Autodesk Fusion 360 part; units mm, degrees
(part 2 of 2)
sketch "Sketch4" plane through (0, 66.2073, 0) normal (0, 1, 0) x (-1, 0, 0)
  line L0 (-39.5671, 5.0322) -> (-39.5671, 0)
  line L1 (-39.5671, 0) -> (-35, 0)
  line L2 (-35, 0) -> (-35, 30)
  line L3 (-35, 30) -> (-45.5671, 30)
  line L4 (-45.5671, 30) -> (-45.5671, 5.0322)
  line L5 (-45.5671, 5.0322) -> (-39.5671, 5.0322)
  line L6 (-39.5671, 5.0322) -> (-19, 5.0322)
  line L7 (-19, 5.0322) -> (-19, 0)
  line L8 (-19, 0) -> (-39.5671, 0)
  line L9 (-39.5671, 0) -> (-39.5671, 5.0322)
  line L10 (-45.5671, 29) -> (-45.5671, 19)
  line L11 (-45.5671, 18.6501) -> (-45.5671, 13.7057)
  line L12 (-45.5671, 13.3545) -> (-45.5671, 9.6128)
  line L13 (-45, 29) -> (-44, 29)
  line L14 (-44, 29) -> (-44, 19)
  line L15 (-44, 19) -> (-45, 19)
  line L16 (-45, 19) -> (-45, 29)
  line L17 (-43.5, 29) -> (-43, 29)
  line L18 (-43, 29) -> (-43, 19)
  line L19 (-43, 19) -> (-43.5, 19)
  line L20 (-43.5, 19) -> (-43.5, 29)
  line L21 (-42.625, 19) -> (-42.625, 29)
  line L22 (-42.125, 29) -> (-42.125, 19)
  line L23 (-42.625, 29) -> (-42.125, 29)
  line L24 (-42.125, 19) -> (-42.625, 19)
  line L25 (-41.75, 19) -> (-41.75, 29)
  line L26 (-41.25, 29) -> (-41.25, 19)
  line L27 (-41.75, 29) -> (-41.25, 29)
  line L28 (-41.25, 19) -> (-41.75, 19)
  line L29 (-40.875, 19) -> (-40.875, 29)
  line L30 (-40.375, 29) -> (-40.375, 19)
  line L31 (-40.875, 29) -> (-40.375, 29)
  line L32 (-40.375, 19) -> (-40.875, 19)
  line L33 (-40, 19) -> (-40, 29)
  line L34 (-39.5, 29) -> (-39.5, 19)
  line L35 (-40, 29) -> (-39.5, 29)
  line L36 (-39.5, 19) -> (-40, 19)
  line L37 (-39.125, 19) -> (-39.125, 29)
  line L38 (-38.625, 29) -> (-38.625, 19)
  line L39 (-39.125, 29) -> (-38.625, 29)
  line L40 (-38.625, 19) -> (-39.125, 19)
  line L41 (-38.25, 19) -> (-38.25, 29)
  line L42 (-37.75, 29) -> (-37.75, 19)
  line L43 (-38.25, 29) -> (-37.75, 29)
  line L44 (-37.75, 19) -> (-38.25, 19)
  line L45 (-37.375, 19) -> (-37.375, 29)
  line L46 (-36.875, 29) -> (-36.875, 19)
  line L47 (-37.375, 29) -> (-36.875, 29)
  line L48 (-36.875, 19) -> (-37.375, 19)
  line L49 (-36.5, 19) -> (-36.5, 29)
  line L50 (-36, 29) -> (-36, 19)
  line L51 (-36.5, 29) -> (-36, 29)
  line L52 (-36, 19) -> (-36.5, 19)
  line L53 (-40.8767, 18.5179) -> (-40.3767, 18.5179)
  line L54 (-40.3767, 18.5179) -> (-40.3767, 10.3968)
  line L55 (-40.3767, 10.3968) -> (-40.8767, 10.3968)
  line L56 (-40.8767, 10.3968) -> (-40.8767, 18.5179)
  line L57 (-39.4967, 18.5179) -> (-39.4967, 10.3968)
  line L58 (-39.9967, 10.3968) -> (-39.9967, 18.5179)
  line L59 (-39.9967, 18.5179) -> (-39.4967, 18.5179)
  line L60 (-39.4967, 10.3968) -> (-39.9967, 10.3968)
  line L61 (-38.6167, 18.5179) -> (-38.6167, 10.3968)
  line L62 (-39.1167, 10.3968) -> (-39.1167, 18.5179)
  line L63 (-39.1167, 18.5179) -> (-38.6167, 18.5179)
  line L64 (-38.6167, 10.3968) -> (-39.1167, 10.3968)
  line L65 (-37.7367, 18.5179) -> (-37.7367, 10.3968)
  line L66 (-38.2367, 10.3968) -> (-38.2367, 18.5179)
  line L67 (-38.2367, 18.5179) -> (-37.7367, 18.5179)
  line L68 (-37.7367, 10.3968) -> (-38.2367, 10.3968)
  line L69 (-36.8567, 18.5179) -> (-36.8567, 10.3968)
  line L70 (-37.3567, 10.3968) -> (-37.3567, 18.5179)
  line L71 (-37.3567, 18.5179) -> (-36.8567, 18.5179)
  line L72 (-36.8567, 10.3968) -> (-37.3567, 10.3968)
  line L73 (-35.9767, 18.5179) -> (-35.9767, 10.3968)
  line L74 (-36.4767, 10.3968) -> (-36.4767, 18.5179)
  line L75 (-36.4767, 18.5179) -> (-35.9767, 18.5179)
  line L76 (-35.9767, 10.3968) -> (-36.4767, 10.3968)
  line L77 (-35.0392, 18.5179) -> (-35.0392, 10.3968)
  line L78 (-35.5392, 10.3968) -> (-35.5392, 18.5179)
  line L79 (-35.5392, 18.5179) -> (-35.0392, 18.5179)
  line L80 (-35.0392, 10.3968) -> (-35.5392, 10.3968)
  line L81 (-34.1017, 18.5179) -> (-34.1017, 10.3968)
  line L82 (-34.6017, 10.3968) -> (-34.6017, 18.5179)
  line L83 (-34.6017, 18.5179) -> (-34.1017, 18.5179)
  line L84 (-34.1017, 10.3968) -> (-34.6017, 10.3968)
  line L85 (-33.1642, 18.5179) -> (-33.1642, 10.3968)
  line L86 (-33.6642, 10.3968) -> (-33.6642, 18.5179)
  line L87 (-33.6642, 18.5179) -> (-33.1642, 18.5179)
  line L88 (-33.1642, 10.3968) -> (-33.6642, 10.3968)
  line L89 (-32.2267, 18.5179) -> (-32.2267, 10.3968)
  line L90 (-32.7267, 10.3968) -> (-32.7267, 18.5179)
  line L91 (-32.7267, 18.5179) -> (-32.2267, 18.5179)
  line L92 (-32.2267, 10.3968) -> (-32.7267, 10.3968)
  line L93 (-31.2892, 18.5179) -> (-31.2892, 10.3968)
  line L94 (-31.7892, 10.3968) -> (-31.7892, 18.5179)
  line L95 (-31.7892, 18.5179) -> (-31.2892, 18.5179)
  line L96 (-31.2892, 10.3968) -> (-31.7892, 10.3968)
  line L97 (-30.3517, 18.5179) -> (-30.3517, 10.3968)
  line L98 (-30.8517, 10.3968) -> (-30.8517, 18.5179)
  line L99 (-30.8517, 18.5179) -> (-30.3517, 18.5179)
  line L100 (-30.3517, 10.3968) -> (-30.8517, 10.3968)
  line L101 (-29.4142, 18.5179) -> (-29.4142, 10.3968)
  line L102 (-29.9142, 10.3968) -> (-29.9142, 18.5179)
  line L103 (-29.9142, 18.5179) -> (-29.4142, 18.5179)
  line L104 (-29.4142, 10.3968) -> (-29.9142, 10.3968)
  line L105 (-28.4767, 18.5179) -> (-28.4767, 10.3968)
  line L106 (-28.9767, 10.3968) -> (-28.9767, 18.5179)
  line L107 (-28.9767, 18.5179) -> (-28.4767, 18.5179)
  line L108 (-28.4767, 10.3968) -> (-28.9767, 10.3968)
  line L109 (-27.5392, 18.5179) -> (-27.5392, 10.3968)
  line L110 (-28.0392, 10.3968) -> (-28.0392, 18.5179)
  line L111 (-28.0392, 18.5179) -> (-27.5392, 18.5179)
  line L112 (-27.5392, 10.3968) -> (-28.0392, 10.3968)
  line L113 (-26.6017, 18.5179) -> (-26.6017, 10.3968)
  line L114 (-27.1017, 10.3968) -> (-27.1017, 18.5179)
  line L115 (-27.1017, 18.5179) -> (-26.6017, 18.5179)
  line L116 (-26.6017, 10.3968) -> (-27.1017, 10.3968)
  line L117 (-25.6642, 18.5179) -> (-25.6642, 10.3968)
  line L118 (-26.1642, 10.3968) -> (-26.1642, 18.5179)
  line L119 (-26.1642, 18.5179) -> (-25.6642, 18.5179)
  line L120 (-25.6642, 10.3968) -> (-26.1642, 10.3968)
  line L121 (-24.7267, 18.5179) -> (-24.7267, 10.3968)
  line L122 (-25.2267, 10.3968) -> (-25.2267, 18.5179)
  line L123 (-25.2267, 18.5179) -> (-24.7267, 18.5179)
  line L124 (-24.7267, 10.3968) -> (-25.2267, 10.3968)
  line L125 (-23.7892, 18.5179) -> (-23.7892, 10.3968)
  line L126 (-24.2892, 10.3968) -> (-24.2892, 18.5179)
  line L127 (-24.2892, 18.5179) -> (-23.7892, 18.5179)
  line L128 (-23.7892, 10.3968) -> (-24.2892, 10.3968)
  line L129 (-22.8517, 18.5179) -> (-22.8517, 10.3968)
  line L130 (-23.3517, 10.3968) -> (-23.3517, 18.5179)
  line L131 (-23.3517, 18.5179) -> (-22.8517, 18.5179)
  line L132 (-22.8517, 10.3968) -> (-23.3517, 10.3968)
  line L133 (-21.9142, 18.5179) -> (-21.9142, 10.3968)
  line L134 (-22.4142, 10.3968) -> (-22.4142, 18.5179)
  line L135 (-22.4142, 18.5179) -> (-21.9142, 18.5179)
  line L136 (-21.9142, 10.3968) -> (-22.4142, 10.3968)
  line L137 (-20.9767, 18.5179) -> (-20.9767, 10.3968)
  line L138 (-21.4767, 10.3968) -> (-21.4767, 18.5179)
  line L139 (-21.4767, 18.5179) -> (-20.9767, 18.5179)
  line L140 (-20.9767, 10.3968) -> (-21.4767, 10.3968)
  line L141 (-40.8858, 9.4833) -> (-40.3858, 9.4833)
  line L142 (-40.3858, 9.4833) -> (-40.3858, 5.4766)
  line L143 (-40.3858, 5.4766) -> (-40.8858, 5.4766)
  line L144 (-40.8858, 5.4766) -> (-40.8858, 9.4833)
  line L145 (-39.962, 5.4766) -> (-39.962, 9.4833)
  line L146 (-39.462, 9.4833) -> (-39.462, 5.4766)
  line L147 (-39.962, 9.4833) -> (-39.462, 9.4833)
  line L148 (-39.462, 5.4766) -> (-39.962, 5.4766)
  line L149 (-39.0382, 5.4766) -> (-39.0382, 9.4833)
  line L150 (-38.5382, 9.4833) -> (-38.5382, 5.4766)
  line L151 (-39.0382, 9.4833) -> (-38.5382, 9.4833)
  line L152 (-38.5382, 5.4766) -> (-39.0382, 5.4766)
  line L153 (-38.1144, 5.4766) -> (-38.1144, 9.4833)
  line L154 (-37.6144, 9.4833) -> (-37.6144, 5.4766)
  line L155 (-38.1144, 9.4833) -> (-37.6144, 9.4833)
  line L156 (-37.6144, 5.4766) -> (-38.1144, 5.4766)
  line L157 (-37.1906, 5.4766) -> (-37.1906, 9.4833)
  line L158 (-36.6906, 9.4833) -> (-36.6906, 5.4766)
  line L159 (-37.1906, 9.4833) -> (-36.6906, 9.4833)
  line L160 (-36.6906, 5.4766) -> (-37.1906, 5.4766)
  line L161 (-36.2668, 5.4766) -> (-36.2668, 9.4833)
  line L162 (-35.7668, 9.4833) -> (-35.7668, 5.4766)
  line L163 (-36.2668, 9.4833) -> (-35.7668, 9.4833)
  line L164 (-35.7668, 5.4766) -> (-36.2668, 5.4766)
  line L165 (-35.343, 5.4766) -> (-35.343, 9.4833)
  line L166 (-34.843, 9.4833) -> (-34.843, 5.4766)
  line L167 (-35.343, 9.4833) -> (-34.843, 9.4833)
  line L168 (-34.843, 5.4766) -> (-35.343, 5.4766)
  line L169 (-34.4192, 5.4766) -> (-34.4192, 9.4833)
  line L170 (-33.9192, 9.4833) -> (-33.9192, 5.4766)
  line L171 (-34.4192, 9.4833) -> (-33.9192, 9.4833)
  line L172 (-33.9192, 5.4766) -> (-34.4192, 5.4766)
  line L173 (-33.4954, 5.4766) -> (-33.4954, 9.4833)
  line L174 (-32.9954, 9.4833) -> (-32.9954, 5.4766)
  line L175 (-33.4954, 9.4833) -> (-32.9954, 9.4833)
  line L176 (-32.9954, 5.4766) -> (-33.4954, 5.4766)
  line L177 (-32.5715, 5.4766) -> (-32.5715, 9.4833)
  line L178 (-32.0715, 9.4833) -> (-32.0715, 5.4766)
  line L179 (-32.5715, 9.4833) -> (-32.0715, 9.4833)
  line L180 (-32.0715, 5.4766) -> (-32.5715, 5.4766)
  line L181 (-31.6477, 5.4766) -> (-31.6477, 9.4833)
  line L182 (-31.1477, 9.4833) -> (-31.1477, 5.4766)
  line L183 (-31.6477, 9.4833) -> (-31.1477, 9.4833)
  line L184 (-31.1477, 5.4766) -> (-31.6477, 5.4766)
  line L185 (-30.7239, 5.4766) -> (-30.7239, 9.4833)
  line L186 (-30.2239, 9.4833) -> (-30.2239, 5.4766)
  line L187 (-30.7239, 9.4833) -> (-30.2239, 9.4833)
  line L188 (-30.2239, 5.4766) -> (-30.7239, 5.4766)
  line L189 (-29.8001, 5.4766) -> (-29.8001, 9.4833)
  line L190 (-29.3001, 9.4833) -> (-29.3001, 5.4766)
  line L191 (-29.8001, 9.4833) -> (-29.3001, 9.4833)
  line L192 (-29.3001, 5.4766) -> (-29.8001, 5.4766)
  line L193 (-28.8763, 5.4766) -> (-28.8763, 9.4833)
  line L194 (-28.3763, 9.4833) -> (-28.3763, 5.4766)
  line L195 (-28.8763, 9.4833) -> (-28.3763, 9.4833)
  line L196 (-28.3763, 5.4766) -> (-28.8763, 5.4766)
  line L197 (-27.9525, 5.4766) -> (-27.9525, 9.4833)
  line L198 (-27.4525, 9.4833) -> (-27.4525, 5.4766)
  line L199 (-27.9525, 9.4833) -> (-27.4525, 9.4833)
  line L200 (-27.4525, 5.4766) -> (-27.9525, 5.4766)
  line L201 (-27.0287, 5.4766) -> (-27.0287, 9.4833)
  line L202 (-26.5287, 9.4833) -> (-26.5287, 5.4766)
  line L203 (-27.0287, 9.4833) -> (-26.5287, 9.4833)
  line L204 (-26.5287, 5.4766) -> (-27.0287, 5.4766)
  line L205 (-26.1049, 5.4766) -> (-26.1049, 9.4833)
  line L206 (-25.6049, 9.4833) -> (-25.6049, 5.4766)
  line L207 (-26.1049, 9.4833) -> (-25.6049, 9.4833)
  line L208 (-25.6049, 5.4766) -> (-26.1049, 5.4766)
  line L209 (-25.1811, 5.4766) -> (-25.1811, 9.4833)
  line L210 (-24.6811, 9.4833) -> (-24.6811, 5.4766)
  line L211 (-25.1811, 9.4833) -> (-24.6811, 9.4833)
  line L212 (-24.6811, 5.4766) -> (-25.1811, 5.4766)
  line L213 (-24.2573, 5.4766) -> (-24.2573, 9.4833)
  line L214 (-23.7573, 9.4833) -> (-23.7573, 5.4766)
  line L215 (-24.2573, 9.4833) -> (-23.7573, 9.4833)
  line L216 (-23.7573, 5.4766) -> (-24.2573, 5.4766)
  line L217 (-23.3335, 5.4766) -> (-23.3335, 9.4833)
  line L218 (-22.8335, 9.4833) -> (-22.8335, 5.4766)
  line L219 (-23.3335, 9.4833) -> (-22.8335, 9.4833)
  line L220 (-22.8335, 5.4766) -> (-23.3335, 5.4766)
  line L221 (-22.4096, 5.4766) -> (-22.4096, 9.4833)
  line L222 (-21.9096, 9.4833) -> (-21.9096, 5.4766)
  line L223 (-22.4096, 9.4833) -> (-21.9096, 9.4833)
  line L224 (-21.9096, 5.4766) -> (-22.4096, 5.4766)
  line L225 (-21.4858, 5.4766) -> (-21.4858, 9.4833)
  line L226 (-20.9858, 9.4833) -> (-20.9858, 5.4766)
  line L227 (-21.4858, 9.4833) -> (-20.9858, 9.4833)
  line L228 (-20.9858, 5.4766) -> (-21.4858, 5.4766)
  line L229 (-27.1017, 19) -> (-26.6017, 19)
  line L230 (-26.6017, 19) -> (-26.6017, 26.1587)
  line L231 (-26.6017, 26.1587) -> (-27.1017, 26.1587)
  line L232 (-27.1017, 26.1587) -> (-27.1017, 19)
  line L233 (-26.1634, 26.1587) -> (-26.1634, 19)
  line L234 (-25.6634, 26.1587) -> (-26.1634, 26.1587)
  line L235 (-25.6634, 19) -> (-25.6634, 26.1587)
  line L236 (-26.1634, 19) -> (-25.6634, 19)
  line L237 (-25.2251, 26.1587) -> (-25.2251, 19)
  line L238 (-24.7251, 26.1587) -> (-25.2251, 26.1587)
  line L239 (-24.7251, 19) -> (-24.7251, 26.1587)
  line L240 (-25.2251, 19) -> (-24.7251, 19)
  line L241 (-24.2867, 26.1587) -> (-24.2867, 19)
  line L242 (-23.7867, 26.1587) -> (-24.2867, 26.1587)
  line L243 (-23.7867, 19) -> (-23.7867, 26.1587)
  line L244 (-24.2867, 19) -> (-23.7867, 19)
  line L245 (-23.3484, 26.1587) -> (-23.3484, 19)
  line L246 (-22.8484, 26.1587) -> (-23.3484, 26.1587)
  line L247 (-22.8484, 19) -> (-22.8484, 26.1587)
  line L248 (-23.3484, 19) -> (-22.8484, 19)
  line L249 (-22.4101, 26.1587) -> (-22.4101, 19)
  line L250 (-21.9101, 26.1587) -> (-22.4101, 26.1587)
  line L251 (-21.9101, 19) -> (-21.9101, 26.1587)
  line L252 (-22.4101, 19) -> (-21.9101, 19)
  line L253 (-21.4717, 26.1587) -> (-21.4717, 19)
  line L254 (-20.9717, 26.1587) -> (-21.4717, 26.1587)
  line L255 (-20.9717, 19) -> (-20.9717, 26.1587)
  line L256 (-21.4717, 19) -> (-20.9717, 19)
  dimension "d69" = 7
  dimension "d70" = 0
  dimension "d71" = 0.5
  dimension "d74" = 4.4
  dimension "d75" = 0
  dimension "d78" = 15
  dimension "d79" = 0
  dimension "d84" = 0.5
  dimension "d87" = 19.4
  dimension "d88" = 0
  dimension "d89" = 0.5
  dimension "d92" = 5.63
  dimension "d93" = 0
  constraint horizontal L6
  constraint vertical L7
  constraint horizontal L8
  constraint vertical L9
  constraint coincident L0.start L5.end
  constraint horizontal L13
  constraint vertical L14
  constraint horizontal L15
  constraint vertical L16
  constraint horizontal L17
  constraint vertical L18
  constraint horizontal L19
  constraint vertical L20
  constraint horizontal L53
  constraint vertical L54
  constraint horizontal L55
  constraint vertical L56
  constraint horizontal L141
  constraint vertical L142
  constraint horizontal L143
  constraint vertical L144
  constraint horizontal L229
  constraint vertical L230
  constraint horizontal L231
  constraint vertical L232
  measures "d71" distance of L53.start L53.end
  measures "d84" distance of L141.start L141.end
  measures "d89" distance of L229.start L229.end
extrude "Extrude12" cut sketch "Sketch4" against normal blind 4 contours L2 L6 L7 L8 bodies 2 6 7
extrude "Extrude13" add sketch "Sketch1" along normal blind 5.032 separate body contours L2 L5 L11 | L2 L5 L6 L10 L11 | L2 L11 L12 | L2 L6 L12 L13 | L5 L6 L10 L13 makes body 9
extrude "Extrude14" cut sketch "Sketch1" along normal blind 5.032 contours L2 L5 L11 bodies 9
sketch "Sketch5" plane through (-8.1042, 3.5534, 0) normal (-0.915834, 0.401558, 0) x (-0.401558, -0.915834, 0)
  line L0 (-67.4977, 5.0322) -> (-67.4977, 0)
  line L1 (-67.4977, 0) -> (-25.8277, 0)
  line L2 (-25.8277, 0) -> (-25.8277, 27)
  line L3 (-25.8277, 27) -> (-68.4119, 27)
  line L4 (-68.4119, 27) -> (-68.4119, 5.0322)
  line L5 (-68.4119, 5.0322) -> (-67.4977, 5.0322)
  line L6 (-49, 10.3833) -> (-45, 10.3833)
  line L7 (-45, 10.3833) -> (-45, 0)
  line L8 (-45, 0) -> (-49, 0)
  line L9 (-49, 0) -> (-49, 10.3833)
  line L10 (-55, 3) -> (-52, 3)
  line L11 (-52, 3) -> (-52, 0)
  line L12 (-52, 0) -> (-55, 0)
  line L13 (-55, 0) -> (-55, 3)
  line L14 (-60, 3) -> (-57, 3)
  line L15 (-57, 3) -> (-57, 0)
  line L16 (-57, 0) -> (-60, 0)
  line L17 (-60, 0) -> (-60, 3)
  line L18 (-65, 3) -> (-63, 3)
  line L19 (-63, 3) -> (-63, 0)
  line L20 (-63, 0) -> (-65, 0)
  line L21 (-65, 0) -> (-65, 3)
  line L22 (-42, 3) -> (-40, 3)
  line L23 (-40, 3) -> (-40, 0)
  line L24 (-40, 0) -> (-42, 0)
  line L25 (-42, 0) -> (-42, 3)
  line L26 (-37, 3) -> (-33, 3)
  line L27 (-33, 3) -> (-33, 0)
  line L28 (-33, 0) -> (-37, 0)
  line L29 (-37, 0) -> (-37, 3)
  line L30 (-30, 3) -> (-28, 3)
  line L31 (-28, 3) -> (-28, 0)
  line L32 (-28, 0) -> (-30, 0)
  line L33 (-30, 0) -> (-30, 3)
  line L34 (-38.3227, 15.6501) -> (-38.3227, 10.7057)
  line L35 (-40.5194, 6.6128) -> (-41.0194, 6.6128)
  line L36 (-39.4151, 6.6128) -> (-39.9151, 6.6128)
  line L37 (-35.0116, 10.7057) -> (-35.5116, 10.7057)
  line L38 (-33.8937, 6.6128) -> (-34.3937, 6.6128)
  line L39 (-35.498, 6.6128) -> (-35.498, 10.3545)
  line L40 (-29.9931, 10.7057) -> (-29.9931, 15.6501)
  line L41 (-34.998, 6.6128) -> (-35.498, 6.6128)
  line L42 (-38.8108, 6.6128) -> (-38.8108, 10.3545)
  line L43 (-36.1153, 10.7057) -> (-36.6153, 10.7057)
  line L44 (-37.7066, 6.6128) -> (-37.7066, 10.3545)
  line L45 (-37.219, 15.6501) -> (-37.219, 10.7057)
  line L46 (-33.2894, 6.6128) -> (-33.2894, 10.3545)
  line L47 (-36.6023, 6.6128) -> (-36.6023, 10.3545)
  line L48 (-41.0345, 26) -> (-40.5345, 26)
  line L49 (-37.7241, 16) -> (-37.7241, 26)
  line L50 (-29.4766, 10.3545) -> (-29.4766, 6.6128)
  line L51 (-40.5345, 16) -> (-41.0345, 16)
  line L52 (-39.431, 16) -> (-39.931, 16)
  line L53 (-40.5301, 10.7057) -> (-41.0301, 10.7057)
  line L54 (-29.4766, 6.6128) -> (-29.9766, 6.6128)
  line L55 (-41.0345, 16) -> (-41.0345, 26)
  line L56 (-31.0808, 10.3545) -> (-30.5808, 10.3545)
  line L57 (-32.1851, 6.6128) -> (-32.1851, 10.3545)
  line L58 (-30.5808, 10.3545) -> (-30.5808, 6.6128)
  line L59 (-42.1379, 26) -> (-41.6379, 26)
  line L60 (-41.6338, 10.7057) -> (-42.1338, 10.7057)
  line L61 (-30, 26) -> (-29.5, 26)
  line L62 (-29.9931, 15.6501) -> (-29.4931, 15.6501)
  line L63 (-36.1153, 15.6501) -> (-36.1153, 10.7057)
  line L64 (-41.0194, 6.6128) -> (-41.0194, 10.3545)
  line L65 (-32.2005, 15.6501) -> (-31.7005, 15.6501)
  line L66 (-41.6237, 6.6128) -> (-42.1237, 6.6128)
  line L67 (-33.3042, 10.7057) -> (-33.3042, 15.6501)
  line L68 (-32.2005, 10.7057) -> (-32.2005, 15.6501)
  line L69 (-42.1237, 6.6128) -> (-42.1237, 10.3545)
  line L70 (-31.0968, 15.6501) -> (-30.5968, 15.6501)
  line L71 (-35.0116, 15.6501) -> (-35.0116, 10.7057)
  line L72 (-33.9079, 15.6501) -> (-33.9079, 10.7057)
  line L73 (-34.4079, 15.6501) -> (-33.9079, 15.6501)
  line L74 (-31.0968, 10.7057) -> (-31.0968, 15.6501)
  line L75 (-33.3042, 15.6501) -> (-32.8042, 15.6501)
  line L76 (-58.688, 6.6128) -> (-58.688, 10.3545)
  line L77 (-40.5194, 10.3545) -> (-40.5194, 6.6128)
  line L78 (-59.7923, 6.6128) -> (-59.7923, 10.3545)
  line L79 (-46.5408, 6.6128) -> (-46.5408, 10.3545)
  line L80 (-50.958, 6.6128) -> (-50.958, 10.3545)
  line L81 (-59.2923, 10.3545) -> (-59.2923, 6.6128)
  line L82 (-53.7708, 10.3545) -> (-53.7708, 6.6128)
  line L83 (-48.7494, 6.6128) -> (-48.7494, 10.3545)
  line L84 (-47.6451, 6.6128) -> (-47.6451, 10.3545)
  line L85 (-31.7005, 15.6501) -> (-31.7005, 10.7057)
  line L86 (-52.0623, 6.6128) -> (-52.0623, 10.3545)
  line L87 (-29.4931, 10.7057) -> (-29.9931, 10.7057)
  line L88 (-30.5968, 10.7057) -> (-31.0968, 10.7057)
  line L89 (-41.0194, 10.3545) -> (-40.5194, 10.3545)
  line L90 (-53.7708, 6.6128) -> (-54.2708, 6.6128)
  line L91 (-39.431, 26) -> (-39.431, 16)
  line L92 (-52.6666, 6.6128) -> (-53.1666, 6.6128)
  line L93 (-49.8537, 6.6128) -> (-49.8537, 10.3545)
  line L94 (-32.7894, 6.6128) -> (-33.2894, 6.6128)
  line L95 (-38.8276, 16) -> (-38.8276, 26)
  line L96 (-57.0837, 6.6128) -> (-57.5837, 6.6128)
  line L97 (-54.8751, 6.6128) -> (-55.3751, 6.6128)
  line L98 (-38.8276, 26) -> (-38.3276, 26)
  line L99 (-35.5172, 26) -> (-35.0172, 26)
  line L100 (-53.1666, 6.6128) -> (-53.1666, 10.3545)
  line L101 (-49.3537, 6.6128) -> (-49.8537, 6.6128)
  line L102 (-42.1379, 16) -> (-42.1379, 26)
  line L103 (-31.6851, 6.6128) -> (-32.1851, 6.6128)
  line L104 (-65, 16) -> (-65, 26)
  line L105 (-53.7746, 10.7057) -> (-54.2746, 10.7057)
  line L106 (-60.8966, 10.7057) -> (-60.8966, 15.6501)
  line L107 (-57.5837, 10.3545) -> (-57.0837, 10.3545)
  line L108 (-58.688, 10.3545) -> (-58.188, 10.3545)
  line L109 (-60.8966, 10.3545) -> (-60.3966, 10.3545)
  line L110 (-55.982, 10.7057) -> (-56.482, 10.7057)
  line L111 (-58.1894, 15.6501) -> (-58.1894, 10.7057)
  line L112 (-54.8783, 10.7057) -> (-55.3783, 10.7057)
  line L113 (-59.7931, 15.6501) -> (-59.2931, 15.6501)
  line L114 (-57.0857, 10.7057) -> (-57.5857, 10.7057)
  line L115 (-47.1451, 6.6128) -> (-47.6451, 6.6128)
  line L116 (-33.9138, 16) -> (-34.4138, 16)
  line L117 (-32.2069, 26) -> (-31.7069, 26)
  line L118 (-57.0837, 10.3545) -> (-57.0837, 6.6128)
  line L119 (-50.458, 6.6128) -> (-50.958, 6.6128)
  line L120 (-43.8323, 10.3545) -> (-43.8323, 6.6128)
  line L121 (-31.1034, 16) -> (-31.1034, 26)
  line L122 (-31.1034, 26) -> (-30.6034, 26)
  line L123 (-55.9794, 10.3545) -> (-55.9794, 6.6128)
  line L124 (-51.5623, 6.6128) -> (-52.0623, 6.6128)
  line L125 (-45.4366, 6.6128) -> (-45.4366, 10.3545)
  line L126 (-48.2494, 6.6128) -> (-48.7494, 6.6128)
  line L127 (-55.9794, 6.6128) -> (-56.4794, 6.6128)
  line L128 (-34.4138, 16) -> (-34.4138, 26)
  line L129 (-54.2708, 10.3545) -> (-53.7708, 10.3545)
  line L130 (-55.3783, 10.7057) -> (-55.3783, 15.6501)
  line L131 (-60.3966, 10.7057) -> (-60.8966, 10.7057)
  line L132 (-56.482, 15.6501) -> (-55.982, 15.6501)
  line L133 (-59.7931, 10.7057) -> (-59.7931, 15.6501)
  line L134 (-33.9138, 26) -> (-33.9138, 16)
  line L135 (-35.5172, 16) -> (-35.5172, 26)
  line L136 (-36.6207, 16) -> (-36.6207, 26)
  line L137 (-30, 16) -> (-30, 26)
  line L138 (-41.0301, 10.7057) -> (-41.0301, 15.6501)
  line L139 (-32.2069, 16) -> (-32.2069, 26)
  line L140 (-30.6034, 26) -> (-30.6034, 16)
  line L141 (-41.0301, 15.6501) -> (-40.5301, 15.6501)
  line L142 (-32.8103, 26) -> (-32.8103, 16)
  line L143 (-36.6207, 26) -> (-36.1207, 26)
  line L144 (-33.3103, 26) -> (-32.8103, 26)
  line L145 (-31.7069, 26) -> (-31.7069, 16)
  line L146 (-29.5, 26) -> (-29.5, 16)
  line L147 (-37.7241, 26) -> (-37.2241, 26)
  line L148 (-59.7923, 10.3545) -> (-59.2923, 10.3545)
  line L149 (-46.0408, 6.6128) -> (-46.5408, 6.6128)
  line L150 (-54.8751, 10.3545) -> (-54.8751, 6.6128)
  line L151 (-56.4794, 6.6128) -> (-56.4794, 10.3545)
  line L152 (-60.3966, 6.6128) -> (-60.8966, 6.6128)
  line L153 (-29.9766, 6.6128) -> (-29.9766, 10.3545)
  line L154 (-36.1023, 6.6128) -> (-36.6023, 6.6128)
  line L155 (-57.5837, 6.6128) -> (-57.5837, 10.3545)
  line L156 (-60.3966, 15.6501) -> (-60.3966, 10.7057)
  line L157 (-55.3793, 26) -> (-54.8793, 26)
  line L158 (-57.5857, 15.6501) -> (-57.0857, 15.6501)
  line L159 (-57.5857, 10.7057) -> (-57.5857, 15.6501)
  line L160 (-58.6894, 15.6501) -> (-58.1894, 15.6501)
  line L161 (-58.6894, 10.7057) -> (-58.6894, 15.6501)
  line L162 (-59.2931, 15.6501) -> (-59.2931, 10.7057)
  line L163 (-56.4828, 26) -> (-55.9828, 26)
  line L164 (-57.5862, 26) -> (-57.0862, 26)
  line L165 (-65, 26) -> (-63, 26)
  line L166 (-52.0623, 10.3545) -> (-51.5623, 10.3545)
  line L167 (-50.9635, 15.6501) -> (-50.4635, 15.6501)
  line L168 (-63, 16) -> (-65, 16)
  line L169 (-50.9635, 10.7057) -> (-50.9635, 15.6501)
  line L170 (-54.8793, 16) -> (-55.3793, 16)
  line L171 (-55.9828, 26) -> (-55.9828, 16)
  line L172 (-58.1897, 16) -> (-58.6897, 16)
  line L173 (-48.2561, 10.7057) -> (-48.7561, 10.7057)
  line L174 (-49.8598, 10.7057) -> (-49.8598, 15.6501)
  line L175 (-57.0862, 16) -> (-57.5862, 16)
  line L176 (-59.2931, 26) -> (-59.2931, 16)
  line L177 (-53.7759, 16) -> (-54.2759, 16)
  line L178 (-53.1666, 10.3545) -> (-52.6666, 10.3545)
  line L179 (-49.8598, 15.6501) -> (-49.3598, 15.6501)
  line L180 (-42.7375, 15.6501) -> (-42.7375, 10.7057)
  line L181 (-42.1338, 10.7057) -> (-42.1338, 15.6501)
  line L182 (-48.2494, 10.3545) -> (-48.2494, 6.6128)
  line L183 (-49.3537, 10.3545) -> (-49.3537, 6.6128)
  line L184 (-51.5623, 10.3545) -> (-51.5623, 6.6128)
  line L185 (-59.2923, 6.6128) -> (-59.7923, 6.6128)
  line L186 (-58.188, 6.6128) -> (-58.688, 6.6128)
  line L187 (-50.458, 10.3545) -> (-50.458, 6.6128)
  line L188 (-29.5, 16) -> (-30, 16)
  line L189 (-44.9366, 10.3545) -> (-44.9366, 6.6128)
  line L190 (-30.6034, 16) -> (-31.1034, 16)
  line L191 (-47.1451, 10.3545) -> (-47.1451, 6.6128)
  line L192 (-44.3323, 6.6128) -> (-44.3323, 10.3545)
  line L193 (-46.0408, 10.3545) -> (-46.0408, 6.6128)
  line L194 (-37.2066, 10.3545) -> (-37.2066, 6.6128)
  line L195 (-36.6023, 10.3545) -> (-36.1023, 10.3545)
  line L196 (-31.0808, 6.6128) -> (-31.0808, 10.3545)
  line L197 (-36.1207, 16) -> (-36.6207, 16)
  line L198 (-33.2894, 10.3545) -> (-32.7894, 10.3545)
  line L199 (-32.8042, 15.6501) -> (-32.8042, 10.7057)
  line L200 (-39.4264, 10.7057) -> (-39.9264, 10.7057)
  line L201 (-37.2241, 26) -> (-37.2241, 16)
  line L202 (-38.3276, 26) -> (-38.3276, 16)
  line L203 (-39.9151, 10.3545) -> (-39.4151, 10.3545)
  line L204 (-32.8042, 10.7057) -> (-33.3042, 10.7057)
  line L205 (-29.9766, 10.3545) -> (-29.4766, 10.3545)
  line L206 (-30.5968, 15.6501) -> (-30.5968, 10.7057)
  line L207 (-36.6153, 10.7057) -> (-36.6153, 15.6501)
  line L208 (-32.7894, 10.3545) -> (-32.7894, 6.6128)
  line L209 (-35.0172, 16) -> (-35.5172, 16)
  line L210 (-29.4931, 15.6501) -> (-29.4931, 10.7057)
  line L211 (-34.998, 10.3545) -> (-34.998, 6.6128)
  line L212 (-38.8108, 10.3545) -> (-38.3108, 10.3545)
  line L213 (-36.6153, 15.6501) -> (-36.1153, 15.6501)
  line L214 (-35.5116, 10.7057) -> (-35.5116, 15.6501)
  line L215 (-31.7005, 10.7057) -> (-32.2005, 10.7057)
  line L216 (-42.728, 10.3545) -> (-42.728, 6.6128)
  line L217 (-41.6379, 16) -> (-42.1379, 16)
  line L218 (-41.6237, 10.3545) -> (-41.6237, 6.6128)
  line L219 (-42.1237, 10.3545) -> (-41.6237, 10.3545)
  line L220 (-38.3108, 10.3545) -> (-38.3108, 6.6128)
  line L221 (-37.719, 15.6501) -> (-37.219, 15.6501)
  line L222 (-36.1023, 10.3545) -> (-36.1023, 6.6128)
  line L223 (-40.5345, 26) -> (-40.5345, 16)
  line L224 (-30.5808, 6.6128) -> (-31.0808, 6.6128)
  line L225 (-37.7066, 10.3545) -> (-37.2066, 10.3545)
  line L226 (-32.1851, 10.3545) -> (-31.6851, 10.3545)
  line L227 (-39.931, 16) -> (-39.931, 26)
  line L228 (-39.931, 26) -> (-39.431, 26)
  line L229 (-38.3276, 16) -> (-38.8276, 16)
  line L230 (-37.2241, 16) -> (-37.7241, 16)
  line L231 (-39.4151, 10.3545) -> (-39.4151, 6.6128)
  line L232 (-42.7414, 26) -> (-42.7414, 16)
  line L233 (-41.6379, 26) -> (-41.6379, 16)
  line L234 (-36.1207, 26) -> (-36.1207, 16)
  line L235 (-31.6851, 10.3545) -> (-31.6851, 6.6128)
  line L236 (-39.4264, 15.6501) -> (-39.4264, 10.7057)
  line L237 (-52.6666, 10.3545) -> (-52.6666, 6.6128)
  line L238 (-43.228, 6.6128) -> (-43.228, 10.3545)
  line L239 (-60.8966, 6.6128) -> (-60.8966, 10.3545)
  line L240 (-33.9079, 10.7057) -> (-34.4079, 10.7057)
  line L241 (-58.188, 10.3545) -> (-58.188, 6.6128)
  line L242 (-38.8227, 15.6501) -> (-38.3227, 15.6501)
  line L243 (-35.5116, 15.6501) -> (-35.0116, 15.6501)
  line L244 (-55.3751, 6.6128) -> (-55.3751, 10.3545)
  line L245 (-54.2708, 6.6128) -> (-54.2708, 10.3545)
  line L246 (-34.4079, 10.7057) -> (-34.4079, 15.6501)
  line L247 (-37.719, 10.7057) -> (-37.719, 15.6501)
  line L248 (-38.8227, 10.7057) -> (-38.8227, 15.6501)
  line L249 (-42.1338, 15.6501) -> (-41.6338, 15.6501)
  line L250 (-48.7586, 16) -> (-48.7586, 26)
  line L251 (-48.2586, 26) -> (-48.2586, 16)
  line L252 (-46.0517, 26) -> (-46.0517, 16)
  line L253 (-52.069, 16) -> (-52.069, 26)
  line L254 (-52.6724, 16) -> (-53.1724, 16)
  line L255 (-49.3621, 26) -> (-49.3621, 16)
  line L256 (-53.1724, 16) -> (-53.1724, 26)
  line L257 (-45.4483, 16) -> (-45.4483, 26)
  line L258 (-49.8621, 16) -> (-49.8621, 26)
  line L259 (-47.6552, 16) -> (-47.6552, 26)
  line L260 (-48.2586, 16) -> (-48.7586, 16)
  line L261 (-50.4655, 26) -> (-50.4655, 16)
  line L262 (-43.8448, 16) -> (-44.3448, 16)
  line L263 (-51.569, 16) -> (-52.069, 16)
  line L264 (-43.8448, 26) -> (-43.8448, 16)
  line L265 (-46.5517, 16) -> (-46.5517, 26)
  line L266 (-46.0517, 16) -> (-46.5517, 16)
  line L267 (-43.228, 10.3545) -> (-42.728, 10.3545)
  line L268 (-44.9483, 26) -> (-44.9483, 16)
  line L269 (-44.3448, 16) -> (-44.3448, 26)
  line L270 (-47.1552, 16) -> (-47.6552, 16)
  line L271 (-44.9483, 16) -> (-45.4483, 16)
  line L272 (-44.9366, 6.6128) -> (-45.4366, 6.6128)
  line L273 (-42.7375, 10.7057) -> (-43.2375, 10.7057)
  line L274 (-50.4655, 16) -> (-50.9655, 16)
  line L275 (-43.2375, 15.6501) -> (-42.7375, 15.6501)
  line L276 (-49.3621, 16) -> (-49.8621, 16)
  line L277 (-51.569, 26) -> (-51.569, 16)
  line L278 (-47.1552, 26) -> (-47.1552, 16)
  line L279 (-50.9655, 16) -> (-50.9655, 26)
  line L280 (-42.7414, 16) -> (-43.2414, 16)
  line L281 (-60.3966, 10.3545) -> (-60.3966, 6.6128)
  line L282 (-34.3937, 6.6128) -> (-34.3937, 10.3545)
  line L283 (-52.6724, 26) -> (-52.6724, 16)
  line L284 (-43.8323, 6.6128) -> (-44.3323, 6.6128)
  line L285 (-42.728, 6.6128) -> (-43.228, 6.6128)
  line L286 (-35.498, 10.3545) -> (-34.998, 10.3545)
  line L287 (-33.8937, 10.3545) -> (-33.8937, 6.6128)
  line L288 (-34.3937, 10.3545) -> (-33.8937, 10.3545)
  line L289 (-31.7069, 16) -> (-32.2069, 16)
  line L290 (-32.8103, 16) -> (-33.3103, 16)
  line L291 (-38.3108, 6.6128) -> (-38.8108, 6.6128)
  line L292 (-40.5301, 15.6501) -> (-40.5301, 10.7057)
  line L293 (-37.2066, 6.6128) -> (-37.7066, 6.6128)
  line L294 (-38.3227, 10.7057) -> (-38.8227, 10.7057)
  line L295 (-33.3103, 16) -> (-33.3103, 26)
  line L296 (-39.9264, 15.6501) -> (-39.4264, 15.6501)
  line L297 (-34.4138, 26) -> (-33.9138, 26)
  line L298 (-41.6338, 15.6501) -> (-41.6338, 10.7057)
  line L299 (-35.0172, 26) -> (-35.0172, 16)
  line L300 (-39.9151, 6.6128) -> (-39.9151, 10.3545)
  line L301 (-39.9264, 10.7057) -> (-39.9264, 15.6501)
  line L302 (-37.219, 10.7057) -> (-37.719, 10.7057)
  line L303 (-49.8621, 26) -> (-49.3621, 26)
  line L304 (-45.4483, 26) -> (-44.9483, 26)
  line L305 (-53.1724, 26) -> (-52.6724, 26)
  line L306 (-52.069, 26) -> (-51.569, 26)
  line L307 (-44.3448, 26) -> (-43.8448, 26)
  line L308 (-44.3323, 10.3545) -> (-43.8323, 10.3545)
  line L309 (-50.9655, 26) -> (-50.4655, 26)
  line L310 (-43.2414, 16) -> (-43.2414, 26)
  line L311 (-46.5517, 26) -> (-46.0517, 26)
  line L312 (-48.7586, 26) -> (-48.2586, 26)
  line L313 (-47.1524, 15.6501) -> (-47.1524, 10.7057)
  line L314 (-47.6552, 26) -> (-47.1552, 26)
  line L315 (-46.0487, 10.7057) -> (-46.5487, 10.7057)
  line L316 (-47.6524, 15.6501) -> (-47.1524, 15.6501)
  line L317 (-44.945, 10.7057) -> (-45.445, 10.7057)
  line L318 (-52.6709, 10.7057) -> (-53.1709, 10.7057)
  line L319 (-49.8537, 10.3545) -> (-49.3537, 10.3545)
  line L320 (-50.958, 10.3545) -> (-50.458, 10.3545)
  line L321 (-53.1709, 10.7057) -> (-53.1709, 15.6501)
  line L322 (-50.4635, 15.6501) -> (-50.4635, 10.7057)
  line L323 (-49.3598, 10.7057) -> (-49.8598, 10.7057)
  line L324 (-48.2561, 15.6501) -> (-48.2561, 10.7057)
  line L325 (-53.1709, 15.6501) -> (-52.6709, 15.6501)
  line L326 (-48.7561, 15.6501) -> (-48.2561, 15.6501)
  line L327 (-50.4635, 10.7057) -> (-50.9635, 10.7057)
  line L328 (-49.3598, 15.6501) -> (-49.3598, 10.7057)
  line L329 (-52.0672, 15.6501) -> (-51.5672, 15.6501)
  line L330 (-51.5672, 15.6501) -> (-51.5672, 10.7057)
  line L331 (-51.5672, 10.7057) -> (-52.0672, 10.7057)
  line L332 (-48.7494, 10.3545) -> (-48.2494, 10.3545)
  line L333 (-48.7561, 10.7057) -> (-48.7561, 15.6501)
  line L334 (-52.6709, 15.6501) -> (-52.6709, 10.7057)
  line L335 (-52.0672, 10.7057) -> (-52.0672, 15.6501)
  line L336 (-45.445, 10.7057) -> (-45.445, 15.6501)
  line L337 (-46.5487, 15.6501) -> (-46.0487, 15.6501)
  line L338 (-47.6451, 10.3545) -> (-47.1451, 10.3545)
  line L339 (-47.6524, 10.7057) -> (-47.6524, 15.6501)
  line L340 (-47.1524, 10.7057) -> (-47.6524, 10.7057)
  line L341 (-46.5408, 10.3545) -> (-46.0408, 10.3545)
  line L342 (-45.445, 15.6501) -> (-44.945, 15.6501)
  line L343 (-44.945, 15.6501) -> (-44.945, 10.7057)
  line L344 (-46.5487, 10.7057) -> (-46.5487, 15.6501)
  line L345 (-43.2375, 10.7057) -> (-43.2375, 15.6501)
  line L346 (-43.8413, 15.6501) -> (-43.8413, 10.7057)
  line L347 (-43.8413, 10.7057) -> (-44.3413, 10.7057)
  line L348 (-43.2414, 26) -> (-42.7414, 26)
  line L349 (-44.3413, 15.6501) -> (-43.8413, 15.6501)
  line L350 (-44.3413, 10.7057) -> (-44.3413, 15.6501)
  line L351 (-46.0487, 15.6501) -> (-46.0487, 10.7057)
  line L352 (-45.4366, 10.3545) -> (-44.9366, 10.3545)
  line L353 (-63, 26) -> (-63, 16)
  line L354 (-61.5, 16) -> (-62, 16)
  line L355 (-58.6897, 16) -> (-58.6897, 26)
  line L356 (-59.2931, 16) -> (-59.7931, 16)
  line L357 (-57.0862, 26) -> (-57.0862, 16)
  line L358 (-60.8966, 16) -> (-60.8966, 26)
  line L359 (-59.7931, 16) -> (-59.7931, 26)
  line L360 (-60.3966, 16) -> (-60.8966, 16)
  line L361 (-60.3966, 26) -> (-60.3966, 16)
  line L362 (-58.1897, 26) -> (-58.1897, 16)
  line L363 (-61.5, 26) -> (-61.5, 16)
  line L364 (-56.4828, 16) -> (-56.4828, 26)
  line L365 (-55.3793, 16) -> (-55.3793, 26)
  line L366 (-57.5862, 16) -> (-57.5862, 26)
  line L367 (-62, 26) -> (-61.5, 26)
  line L368 (-54.2759, 26) -> (-53.7759, 26)
  line L369 (-53.7759, 26) -> (-53.7759, 16)
  line L370 (-54.2759, 16) -> (-54.2759, 26)
  line L371 (-54.8793, 26) -> (-54.8793, 16)
  line L372 (-62, 16) -> (-62, 26)
  line L373 (-55.9828, 16) -> (-56.4828, 16)
  line L374 (-58.6897, 26) -> (-58.1897, 26)
  line L375 (-60.8966, 26) -> (-60.3966, 26)
  line L376 (-59.7931, 26) -> (-59.2931, 26)
  line L377 (-60.8966, 15.6501) -> (-60.3966, 15.6501)
  line L378 (-54.2746, 15.6501) -> (-53.7746, 15.6501)
  line L379 (-55.3783, 15.6501) -> (-54.8783, 15.6501)
  line L380 (-58.1894, 10.7057) -> (-58.6894, 10.7057)
  line L381 (-56.482, 10.7057) -> (-56.482, 15.6501)
  line L382 (-55.3751, 10.3545) -> (-54.8751, 10.3545)
  line L383 (-53.7746, 15.6501) -> (-53.7746, 10.7057)
  line L384 (-54.8783, 15.6501) -> (-54.8783, 10.7057)
  line L385 (-57.0857, 15.6501) -> (-57.0857, 10.7057)
  line L386 (-59.2931, 10.7057) -> (-59.7931, 10.7057)
  line L387 (-55.982, 15.6501) -> (-55.982, 10.7057)
  line L388 (-56.4794, 10.3545) -> (-55.9794, 10.3545)
  line L389 (-54.2746, 10.7057) -> (-54.2746, 15.6501)
  dimension "d100" = 32
  dimension "d101" = 0
  dimension "d104" = 29.8
  dimension "d105" = 0
  dimension "d108" = 30.92
  dimension "d109" = 0
  dimension "d110" = 0.5
  dimension "d111" = 0.5
  constraint horizontal L6
  constraint vertical L7
  constraint horizontal L8
  constraint vertical L9
  constraint coincident L1 L7.end
  constraint horizontal L10
  constraint vertical L11
  constraint horizontal L12
  constraint vertical L13
  constraint coincident L1 L11.end
  constraint horizontal L14
  constraint vertical L15
  constraint horizontal L16
  constraint vertical L17
  constraint coincident L1 L15.end
  constraint horizontal L18
  constraint vertical L19
  constraint horizontal L20
  constraint vertical L21
  constraint coincident L1 L19.end
  constraint horizontal L22
  constraint vertical L23
  constraint horizontal L24
  constraint vertical L25
  constraint coincident L1 L23.end
  constraint horizontal L26
  constraint vertical L27
  constraint horizontal L28
  constraint vertical L29
  constraint coincident L1 L27.end
  constraint horizontal L30
  constraint vertical L31
  constraint horizontal L32
  constraint vertical L33
  constraint coincident L1 L31.end
  constraint horizontal L165
  constraint vertical L353
  constraint horizontal L168
  constraint vertical L104
  constraint horizontal L367
  constraint vertical L363
  constraint horizontal L354
  constraint vertical L372
  constraint horizontal L377
  constraint vertical L156
  constraint horizontal L131
  constraint vertical L106
  constraint horizontal L113
  constraint vertical L162
  constraint horizontal L386
  constraint vertical L133
  constraint horizontal L109
  constraint vertical L281
  constraint horizontal L152
  constraint vertical L239
  measures "d110" distance of L367.start L363.start
  measures "d111" distance of L106.end L156.start
extrude "Extrude15" cut sketch "Sketch5" against normal blind 3 contours L1 L18 L19 L20 L21 | L1 L14 L15 L16 L17 | L1 L30 L31 L32 L33 | L1 L10 L11 L12 L13 | L1 L26 L27 L28 L29 | L1 L6 L7 L8 L9 L125 L272 L352 | L1 L22 L23 L24 L25 | L7 L125 L272 L352 | L79 L149 L193 L341 | L83 L126 L182 L332 | L84 L115 L191 L338 bodies 2
extrude "Extrude16" cut sketch "Sketch2" against normal blind 1 contours L3 L5 L6 L13 L29 L30 L31 L32 | L0 L13 L21 L22 L23 L24 | L5 L13 L25 L26 L27 L28 bodies 2 5
extrude "Extrude17" cut sketch "Sketch3" against normal blind 2 contours L22 L23 L24 L25 | L26 L27 L28 L29 | L30 L31 L32 L33 | L34 L35 L36 L37 | L38 L39 L40 L41 | L42 L43 L44 L45 | L46 L47 L48 L49 | L50 L51 L52 L53 | L54 L55 L56 L57 | L58 L59 L60 L61 | L62 L63 L64 L65 | L66 L67 L68 L69 | L70 L71 L72 L73 | L74 L75 L76 L77 | L78 L79 L80 L81 | L82 L83 L84 L85 | L86 L87 L88 L89 | L90 L91 L92 L93 | L94 L95 L96 L97 | L98 L99 L100 L101 | L102 L103 L104 L105 | L106 L107 L108 L109 | L110 L111 L112 L113 | L114 L115 L116 L117 | L118 L119 L120 L121 | L122 L123 L124 L125 | L126 L127 L128 L129 | L130 L131 L132 L133 | L134 L135 L136 L137 | L138 L139 L140 L141 | L142 L143 L144 L145 bodies 1
extrude "Extrude18" add sketch "Sketch3" against normal blind 3 contours L22 L23 L24 L25 bodies 1
extrude "Extrude19" cut sketch "Sketch3" against normal blind 1 contours L22 L23 L24 L25 bodies 1
extrude "Extrude20" cut sketch "Sketch3" against normal blind 3 contours L146 L147 L148 L149 | L150 L151 L152 L153 | L154 L155 L156 L157 | L158 L159 L160 L161 | L162 L163 L164 L165 | L166 L167 L168 L169 | L170 L171 L172 L173 | L174 L175 L176 L177 | L178 L179 L180 L181 | L182 L183 L184 L185 | L186 L187 L188 L189 | L190 L191 L192 L193 | L194 L195 L196 L197 | L198 L199 L200 L201 | L202 L203 L204 L205 | L206 L207 L208 L209 | L210 L211 L212 L213 | L214 L215 L216 L217 | L218 L219 L220 L221 | L222 L223 L224 L225 | L226 L227 L228 L229 | L230 L231 L232 L233 | L234 L235 L236 L237 | L238 L239 L240 L241 | L242 L243 L244 L245 | L246 L247 L248 L249 | L250 L251 L252 L253 | L254 L255 L256 L257 | L258 L259 L260 L261 bodies 1
extrude "Extrude21" cut sketch "Sketch3" against normal blind 2 contours L262 L263 L264 L265 | L266 L267 L268 L269 | L270 L271 L272 L273 | L274 L275 L276 L277 | L278 L279 L280 L281 | L282 L283 L284 L285 | L286 L287 L288 L289 | L290 L291 L292 L293 | L294 L295 L296 L297 | L298 L299 L300 L301 | L302 L303 L304 L305 | L306 L307 L308 L309 | L310 L311 L312 L313 | L314 L315 L316 L317 | L318 L319 L320 L321 | L322 L323 L324 L325 | L326 L327 L328 L329 | L330 L331 L332 L333 | L334 L335 L336 L337 | L338 L339 L340 L341 | L342 L343 L344 L345 | L346 L347 L348 L349 | L350 L351 L352 L353 | L354 L355 L356 L357 | L358 L359 L360 L361 | L362 L363 L364 L365 | L366 L367 L368 L369 | L370 L371 L372 L373 | L374 L375 L376 L377 bodies 1
extrude "Extrude22" add sketch "Sketch5" against normal blind 3 contours L1 L18 L19 L20 L21 bodies 2
extrude "Extrude23" cut sketch "Sketch5" against normal blind 0.8 contours L1 L18 L19 L20 L21 bodies 2
extrude "Extrude24" add 1 faces at (19.3311, 62.3525, 3) along direction (0, 0, 1) blind 2.032 on bodies 2 bodies 2
extrude "Extrude25" cut sketch "Sketch4" against normal blind 2 contours L17 L18 L19 L20 | L21 L22 L23 L24 | L25 L26 L27 L28 | L29 L30 L31 L32 | L33 L34 L35 L36 | L37 L38 L39 L40 | L41 L42 L43 L44 | L45 L46 L47 L48 | L49 L50 L51 L52 | L53 L54 L55 L56 | L57 L58 L59 L60 | L61 L62 L63 L64 | L65 L66 L67 L68 | L69 L70 L71 L72 | L73 L74 L75 L76 bodies 1
extrude "Extrude26" cut sketch "Sketch4" against normal blind 1 contours L13 L14 L15 L16 bodies 1
extrude "Extrude27" cut sketch "Sketch4" against normal blind 2 contours L2 L165 L167 L168 | L2 L166 L167 L168 | L17 L18 L19 L20 | L21 L22 L23 L24 | L25 L26 L27 L28 | L29 L30 L31 L32 | L33 L34 L35 L36 | L37 L38 L39 L40 | L41 L42 L43 L44 | L45 L46 L47 L48 | L49 L50 L51 L52 | L53 L54 L55 L56 | L57 L58 L59 L60 | L61 L62 L63 L64 | L65 L66 L67 L68 | L69 L70 L71 L72 | L73 L74 L75 L76 | L77 L78 L79 L80 | L113 L114 L115 L116 | L117 L118 L119 L120 | L121 L122 L123 L124 | L125 L126 L127 L128 | L129 L130 L131 L132 | L133 L134 L135 L136 | L137 L138 L139 L140 | L141 L142 L143 L144 | L145 L146 L147 L148 | L149 L150 L151 L152 | L153 L154 L155 L156 | L157 L158 L159 L160 | L161 L162 L163 L164 | L169 L170 L171 L172 | L173 L174 L175 L176 | L177 L178 L179 L180 | L181 L182 L183 L184 | L185 L186 L187 L188 | L189 L190 L191 L192 | L193 L194 L195 L196 | L197 L198 L199 L200 | L201 L202 L203 L204 | L205 L206 L207 L208 | L209 L210 L211 L212 | L213 L214 L215 L216 | L217 L218 L219 L220 | L221 L222 L223 L224 | L225 L226 L227 L228 | L229 L230 L231 L232 | L233 L234 L235 L236 | L237 L238 L239 L240 | L241 L242 L243 L244 | L245 L246 L247 L248 | L249 L250 L251 L252 | L253 L254 L255 L256 bodies 1 2 7
extrude "Extrude28" add sketch "Sketch4" against normal blind 3.611 contours L77 L78 L79 L80 bodies 1
extrude "Extrude29" cut sketch "Sketch5" against normal blind 2 contours L7 L125 L272 L352 | L7 L189 L272 L352 | L34 L242 L248 L294 | L35 L64 L77 L89 | L36 L203 L231 L300 | L37 L71 L214 L243 | L38 L282 L287 L288 | L39 L41 L211 L286 | L40 L62 L87 L210 | L42 L212 L220 L291 | L43 L63 L207 L213 | L44 L194 L225 L293 | L45 L221 L247 L302 | L46 L94 L198 L208 | L47 L154 L195 L222 | L48 L51 L55 L223 | L49 L147 L201 L230 | L50 L54 L153 L205 | L52 L91 L227 L228 | L53 L138 L141 L292 | L56 L58 L196 L224 | L57 L103 L226 L235 | L59 L102 L217 L233 | L60 L181 L249 L298 | L61 L137 L146 L188 | L65 L68 L85 L215 | L66 L69 L218 L219 | L67 L75 L199 L204 | L70 L74 L88 L206 | L72 L73 L240 L246 | L76 L108 L186 L241 | L78 L81 L148 L185 | L79 L149 L193 L341 | L80 L119 L187 L320 | L82 L90 L129 L245 | L83 L126 L182 L332 | L84 L115 L191 L338 | L86 L124 L166 L184 | L92 L100 L178 L237 | L93 L101 L183 L319 | L95 L98 L202 L229 | L96 L107 L118 L155 | L97 L150 L244 L382 | L99 L135 L209 L299 | L105 L378 L383 L389 | L106 L131 L156 L377 | L109 L152 L239 L281 | L110 L132 L381 L387 | L111 L160 L161 L380 | L112 L130 L379 L384 | L113 L133 L162 L386 | L114 L158 L159 L385 | L116 L128 L134 L297 | L117 L139 L145 L289 | L120 L192 L284 L308 | L121 L122 L140 L190 | L123 L127 L151 L388 | L136 L143 L197 L234 | L142 L144 L290 L295 | L157 L170 L365 L371 | L163 L171 L364 L373 | L164 L175 L357 L366 | L167 L169 L322 L327 | L172 L355 L362 L374 | L173 L324 L326 L333 | L174 L179 L323 L328 | L176 L356 L359 L376 | L177 L368 L369 L370 | L180 L273 L275 L345 | L200 L236 L296 L301 | L216 L238 L267 L285 | L232 L280 L310 L348 | L250 L251 L260 L312 | L252 L265 L266 L311 | L253 L263 L277 L306 | L254 L256 L283 L305 | L255 L258 L276 L303 | L257 L268 L271 L304 | L259 L270 L278 L314 | L261 L274 L279 L309 | L262 L264 L269 L307 | L313 L316 L339 L340 | L315 L337 L344 L351 | L317 L336 L342 L343 | L318 L321 L325 L334 | L329 L330 L331 L335 | L346 L347 L349 L350 | L354 L363 L367 L372 | L358 L360 L361 L375 bodies 2
extrude "Extrude30" add sketch "Sketch5" against normal blind 3 contours L1 L6 L7 L8 L9 L125 L272 L352 | L7 L125 L272 L352 | L7 L189 L272 L352 | L79 L149 L193 L341 | L83 L126 L182 L332 | L84 L115 L191 L338 bodies 2
extrude "Extrude31" cut sketch "Sketch5" against normal blind 2 contours L1 L6 L7 L8 L9 L125 L272 L352 | L7 L125 L272 L352 | L79 L149 L193 L341 | L83 L126 L182 L332 | L84 L115 L191 L338 bodies 2
extrude "Extrude32" cut sketch "Sketch2" against normal blind 2 contours L353 L355 L356 L359 L375 L378 | L357 L360 L361 L365 L386 L387 | L366 L380 L390 L392 L393 L395 | L354 L358 L362 L363 L364 L368 | L376 L384 L385 L388 L389 L394 | L369 L373 L379 L383 L391 L398 | L372 L374 L377 L381 L396 L399 bodies 2
extrude "Extrude33" cut sketch "Sketch2" against normal blind 2 contours L4 L183 L214 L260 | L4 L183 L230 L260 | L4 L200 L232 L249 | L4 L232 L243 L249 | L4 L213 L228 L264 | L4 L193 L213 L228 | L4 L182 L226 L227 | L4 L182 L226 L252 | L4 L177 L219 L259 | L4 L174 L177 L219 | L4 L179 L222 L225 | L4 L179 L222 L223 | L33 L37 L72 L73 | L34 L97 L100 L206 | L35 L86 L90 L147 | L36 L56 L68 L70 | L38 L93 L134 L150 | L39 L40 L115 L121 | L41 L45 L51 L116 | L42 L65 L109 L149 | L43 L62 L103 L148 | L44 L49 L114 L120 | L46 L82 L105 L106 | L47 L50 L113 L118 | L48 L63 L101 L110 | L52 L111 L112 L117 | L53 L55 L59 L66 | L54 L61 L96 L140 | L57 L64 L99 L108 | L58 L69 L71 L74 | L60 L125 L142 L153 | L67 L84 L139 L145 | L75 L136 L156 L163 | L76 L83 L143 L144 | L77 L130 L131 L161 | L78 L126 L132 L154 | L79 L123 L124 L128 | L80 L85 L91 L146 | L81 L98 L102 L119 | L87 L95 L127 L151 | L88 L92 L138 L141 | L89 L104 L122 L152 | L94 L107 L199 L241 | L129 L137 L157 L159 | L133 L155 L158 L162 | L135 L160 L164 L165 | L166 L203 L211 L216 | L167 L169 L236 L238 | L168 L184 L229 L244 | L170 L176 L196 L239 | L171 L209 L234 L255 | L172 L175 L202 L250 | L173 L188 L191 L204 | L178 L197 L205 L246 | L180 L215 L220 L253 | L181 L194 L217 L237 | L185 L186 L235 L258 | L187 L224 L240 L245 | L189 L242 L247 L254 | L190 L210 L257 L263 | L192 L221 L261 L262 | L195 L212 L218 L248 | L198 L201 L207 L251 | L208 L231 L233 L256 | L265 L266 L267 L268 | L269 L270 L271 L272 | L273 L274 L275 L276 | L277 L278 L279 L280 | L281 L282 L283 L284 | L285 L286 L287 L288 | L289 L290 L291 L292 | L293 L294 L295 L296 | L297 L298 L299 L300 | L301 L302 L303 L304 bodies 1 2 5
extrude "Extrude34" cut sketch "Sketch2" against normal blind 2 contours L305 L306 L307 L308 L344 L349 | L309 L310 L311 L312 L342 L352 | L313 L314 L315 L316 L340 L341 | L317 L318 L319 L320 L337 L345 | L321 L322 L323 L324 L347 L351 | L325 L326 L327 L328 L343 L350 | L329 L330 L331 L332 L338 L348 | L333 L334 L335 L336 L339 L346 bodies 1
extrude "Extrude35" add sketch "Sketch2" against normal blind 1.5 contours L5 L13 L25 L26 L27 L28 bodies 2
extrude "Extrude36" cut sketch "Sketch2" against normal blind 1 contours L5 L13 L25 L26 L27 L28 bodies 2
extrude "Extrude37" add sketch "Sketch5" against normal blind 0.8 contours L1 L18 L19 L20 L21 bodies 2
extrude "Extrude38" cut sketch "Sketch5" against normal blind 0.5 contours L1 L18 L19 L20 L21 bodies 2
extrude "Extrude39" add sketch "Sketch1" against normal blind 2 separate body contours L0 L1 L2 L4 L5 L11 L13 | L2 L5 L11 | L1 L5 L6 L7 | L2 L5 L6 L10 L11 | L2 L11 L12 | L5 L11 L13 | L1 L2 L3 L6 L12 L13 | L5 L6 L7 L8 | L2 L6 L12 L13 | L5 L6 L10 L13 | L5 L6 L8 L9 | L5 L6 L9 L13 | L14 L15 L16 L17 L18 | L15 L16 L18 makes body 10
extrude "Extrude40" cut sketch "Sketch1" against normal blind 15 contours L15 L16 L18 bodies 10
extrude "Extrude41" add sketch "Sketch4" against normal blind 2 contours L229 L230 L231 L232 | L233 L234 L235 L236 | L237 L238 L239 L240 bodies 2
extrude "Extrude42" cut sketch "Sketch4" against normal blind 0.5 contours L229 L230 L231 L232 bodies 2
extrude "Extrude43" cut sketch "Sketch4" against normal blind 1 contours L233 L234 L235 L236 bodies 2
extrude "Extrude44" cut sketch "Sketch4" against normal blind 2 contours L237 L238 L239 L240 bodies 2
extrude "Extrude45" add sketch "Sketch4" against normal blind 2 contours L113 L114 L115 L116 | L117 L118 L119 L120 bodies 2
extrude "Extrude46" cut sketch "Sketch4" against normal blind 0.5 contours L113 L114 L115 L116 bodies 2
extrude "Extrude47" cut sketch "Sketch4" against normal blind 1 contours L117 L118 L119 L120 bodies 2
